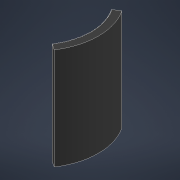
# Autodesk Inventor part: holder3_cushion
Saved by Autodesk Inventor 2021 (Build 250183000, 183)
## iProperties
Created: 2021-06-14
Part Number: holder3_cushion
Material: Rubber
Document SubType Name: Modeling
Designer: Watchdog
Density: 0.93 g/cm^3
Appearance: Rubber - Black
Author: Watchdog
Autodesk Inventor part; units mm, degrees
ref_plane "YZ Plane" through (0, 0, 0) normal (1, 0, 0) x (0, 1, 0)
ref_plane "XZ Plane" through (0, 0, 0) normal (0, 1, 0) x (-1, 0, 0)
ref_plane "XY Plane" through (0, 0, 0) normal (0, 0, 1) x (1, 0, 0)
sketch "Sketch1" plane through (0, 0, 0) normal (0, 1, 0) x (-1, 0, 0)
  arc A0 (-10.133, 6.6732) -> (-10.133, -6.6732) centre (0, 0) ccw
  line L0 (-10.133, -6.6732) -> (-8.8803, -5.8482)
  line L1 (-8.8803, 5.8482) -> (-10.133, 6.6732)
  arc A1 (-8.8803, 5.8482) -> (-8.8803, -5.8482) centre (0, 0) ccw
  point P0 (-12.133, 0)
  dimension "d0" = 12.133
  dimension "d2" = 12.133
  dimension "d3" = 0
  dimension "d5" = 2
  dimension "d6" = 2
  dimension "d7" = 1.5
  constraints: 5 point on circle, 4 end point, 2 centre point, 2 coincident, 2 line through centre
  measures "d0" radius of A0
  measures "d2" distance of point (0, 0) point (-12.133, 0)
  measures "d3" vertical distance of point (0, 0) point (-12.133, 0)
  measures "d5" horizontal distance of point (-12.133, 0) L0.start
  measures "d6" horizontal distance of point (-12.133, 0) L1.end
  measures "d7" radial gap between concentric circles of A0 A1
extrude "Extrusion1" add sketch "Sketch1" along normal blind 20
sketch "Sketch2" plane through (0, 20, 0) normal (0, 1, 0) x (1, 0, 0)
  arc A0 (8.8803, -5.8482) -> (8.8803, 5.8482) centre (0, 0) ccw projected
  arc A1 (9.0178, 5.6338) -> (8.9103, 5.8024) centre (8.9645, 5.7183) ccw
  line L0 (0, 0) -> (10, 0)
  line L1 (10.133, 6.6732) -> (8.8803, 5.8482) projected
  line L2 (0, 0) -> (16.8616, 10.7558)
  dimension "d11" = 0.1
  dimension "d12" = 10
  dimension "d13" = 33.367
  dimension "d14" = 20
  dimension "d15" = 0.834
  constraints: 5 point on circle, 4 end point, 1 centre point, 1 horizontal, 1 point on line
  measures "d11" radius of A1
  measures "d12" distance of L0.start L0.end
  measures "d13" angle of L0 L1
  measures "d14" distance of L0.start L2.end
  measures "d15" angle of L1 L2
extrude "Extrusion2" cut sketch "Sketch2" against normal through all
pattern_circular "Circular Pattern1" count 40 over 66.79 about axis through (0, -10, 0) along (0, -1, 0) of "Extrusion2"
equation "\"d0\" = r"
equation "\"d2\" = d0"
equation "\"d5\" = segment"
equation "\"d6\" = segment"
equation "\"d7\" = t"
equation "\"segment\" = 2"
equation "\"t\" = 1.5"
equation "\"r\" = 12.133"
body "Solid1"
